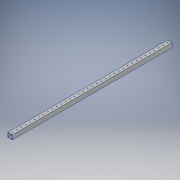
# Autodesk Inventor part: versatubing long boy
Saved by Autodesk Inventor 2018 (Build 220112000, 112)
## iProperties
Created: 2016-07-01
Part Number: versatubing long boy
Material: Aluminum 6061
Document SubType Name: Modeling
Designer: rickab1
Mass: 81.5525 g
Surface Area: 596.561 cm^2
Volume: 30.2046 cm^3
Density: 2.7 g/cm^3
Appearance: Aluminum - Flat
Author: rickab1
Autodesk Inventor part; units mm, degrees
ref_plane "YZ Plane" through (0, 0, 0) normal (1, 0, 0) x (0, 1, 0)
ref_plane "XZ Plane" through (0, 0, 0) normal (0, 1, 0) x (-1, 0, 0)
ref_plane "XY Plane" through (0, 0, 0) normal (0, 0, 1) x (1, 0, 0)
sketch "Sketch1" plane through (0, 0, 0) normal (0, 0, 1) x (1, 0, 0)
  line L0 (-12.7, -12.7) -> (12.7, -12.7)
  line L1 (12.7, -12.7) -> (12.7, 12.7)
  line L2 (12.7, 12.7) -> (-12.7, 12.7)
  line L3 (-12.7, 12.7) -> (-12.7, -12.7)
  line L4 (-12.7, -12.7) -> (12.7, 12.7) construction
  line L5 (12.7, -12.7) -> (-12.7, 12.7) construction
  line L6 (-10.16, 10.16) -> (10.16, 10.16)
  line L7 (10.16, 10.16) -> (10.16, -10.16)
  line L8 (10.16, -10.16) -> (-10.16, -10.16)
  line L9 (-10.16, -10.16) -> (-10.16, 10.16)
  point P0 (0, 0)
  dimension "l1" = 25.4
  dimension "l2" = 25.4
  dimension "wt" = 2.54
  constraints: 20 end point, 4 parallel, 2 midpoint, 2 perpendicular, 1 horizontal, 3 other
  measures "l1" distance of L1.end L2.end
  measures "l2" distance of L2.end L0.start
  measures "wt" distance between parallel lines of L1 L7
extrude "Extrusion1" add sketch "Sketch1" against normal blind 914.4
sketch "Sketch2" plane through (-12.7, 12.7, 0) normal (0, 1, 0) x (1, 0, 0)
  line L0 (25.4, 0) -> (0, 0) projected
  line L1 (25.4, 0) -> (25.4, 914.4) projected
  line L2 (0, 914.4) -> (25.4, 914.4) projected
  line L3 (0, 0) -> (0, 914.4) projected
  point P0 (12.7, 0)
  point P1 (12.7, 12.7)
  dimension "d5" = 25.4
  dimension "d6" = 12.7
  dimension "d7" = 12.7
  measures "d5" distance of L0.start L0.end
  measures "d6" distance from line of L3 point (12.7, 12.7)
  measures "d7" distance from line of L0 point (12.7, 12.7)
hole "Hole3" at (0, 12.7, -12.7) direction (0, -1, 0) diameter 4.0894 end through all
sketch "Sketch3" plane through (12.7, -12.7, 0) normal (1, 0, 0) x (0, 0, -1)
  line L0 (0, 0) -> (0, 25.4) projected
  line L1 (0, 0) -> (914.4, 0) projected
  line L2 (914.4, 25.4) -> (914.4, 0) projected
  line L3 (0, 25.4) -> (914.4, 25.4) projected
  point P0 (0, 12.7)
  point P1 (25.4, 12.7)
  dimension "d22" = 25.4
  dimension "d23" = 12.7
  dimension "d24" = 25.4
  measures "d22" distance of L0.start L0.end
  measures "d23" distance from line of L1 point (25.4, 12.7)
  measures "d24" distance from line of L0 point (25.4, 12.7)
hole "Hole4" [suppressed]
pattern_linear "Rectangular Pattern1" count 37 spacing 25.4 along (0, 0, -1) of "Hole3"
pattern_linear "Rectangular Pattern2" [suppressed]
equation "\"d6\" = 0.5 * d5"
equation "\"d23\" = 0.5 * d22"
body "Solid1"
